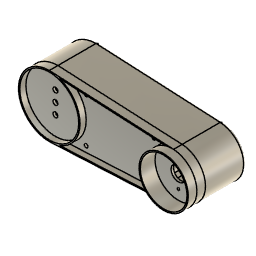
TRARM02_Link3 (Autodesk Fusion 360 design; units mm, degrees)
Autodesk Fusion 360 part; units mm, degrees
sketch "스케치1" plane through (0, 0, 0) normal (0, 0, 1) x (1, 0, 0) in component "TRARM02_Link3A_100x50x7 v1"
  line L0 (19.9753, 100.9938) -> (25, 0)
  line L1 (-19.9753, 100.9938) -> (-25, 0)
  arc A0 (19.9753, 100.9938) -> (-19.9753, 100.9938) centre (0, 100) ccw
  arc A1 (-25, 0) -> (25, 0) centre (0, 0) ccw
  dimension "d1" = 50
  dimension "d222" = 20
  dimension "d223" = 100
  constraint coincident A1.centre origin
  constraint tangent L1 A0
  constraint horizontal A1.centre L1.end
  constraint horizontal A1.centre L0.end
  constraint vertical A1.centre A0.centre
  constraint tangent L0 A0
  measures "d1" diameter of A1
  measures "d222" radius of A0
  measures "d223" distance of A1.centre A0.centre
extrude "돌출1" add sketch "스케치1" along normal blind 2 makes body 1 in component "TRARM02_Link3A_100x50x7 v1"
sketch "스케치2" plane through (0, 0, 2) normal (0, 0, 1) x (-1, 0, 0) in component "TRARM02_Link3A_100x50x7 v1"
  arc A0 (-19.9753, -100.9938) -> (19.9753, -100.9938) centre (0, -100) ccw
  line L0 (19.9753, -100.9938) -> (25, 0)
  line L1 (-25, 0) -> (-19.9753, -100.9938)
  line L2 (19.9753, -100.9938) -> (25, 0)
  arc A1 (-19.9753, -100.9938) -> (19.9753, -100.9938) centre (0, -100) ccw
  line L3 (-25, 0) -> (-19.9753, -100.9938)
  arc A2 (25, 0) -> (-25, 0) centre (0, 0) ccw
  line L4 (-23.5864, -8.2873) -> (-19.2868, -94.7068)
  line L5 (19.2868, -94.7068) -> (23.5864, -8.2873)
  circle A3 centre (0, -100) radius 19
  circle A4 centre (0, 0) radius 23.9691
  arc A5 (-23.5864, -8.2873) -> (23.5864, -8.2873) centre (0, 0) ccw
  arc A6 (25, 0) -> (-25, 0) centre (0, 0) ccw
  arc A7 (-19.9753, -100.9938) -> (19.9753, -100.9938) centre (0, -100) ccw
  arc A8 (19.2868, -94.7068) -> (-19.2868, -94.7068) centre (0, -100) ccw
  constraint concentric A0 A7
  constraint concentric A1 A3
  constraint tangent L4 A3
  constraint concentric A2 A5
  constraint coincident L1.start A5
  constraint concentric A2 A4
  constraint tangent L4 A4
  constraint concentric A5 A6
  constraint coincident L5.start A7
  constraint concentric A7 A8
extrude "돌출25" add sketch "스케치2" along normal blind 5 bodies 1 in component "TRARM02_Link3A_100x50x7 v1"
sketch "스케치22" plane through (0, 0, 2) normal (0, 0, 1) x (-1, 0, 0) in component "TRARM02_Link3A_100x50x7 v1"
  circle A0 centre (0, 0) radius 2
  circle A1 centre (-8.7, 0) radius 2
  circle A2 centre (8.7, 0) radius 2
  circle A3 centre (0, -100) radius 6
  circle A4 centre (-11, -100) radius 1
  circle A5 centre (11, -100) radius 1
  dimension "d208" = 4
  dimension "d209" = 8.7
  dimension "d210" = 8.7
  dimension "d226" = 12
  dimension "d227" = 2
  dimension "d228" = 11
  dimension "d229" = 11
  dimension "d230" = 100
  constraint coincident A0.centre origin
  constraint equal A0 A2
  constraint equal A0 A1
  constraint horizontal A0.centre A1.centre
  constraint horizontal A0.centre A2.centre
  constraint equal A4 A5
  constraint horizontal A3.centre A5.centre
  constraint horizontal A3.centre A4.centre
  constraint vertical A0.centre A3.centre
  measures "d208" diameter of A0
  measures "d209" distance of A0.centre A1.centre
  measures "d210" distance of A0.centre A2.centre
  measures "d226" diameter of A3
  measures "d227" diameter of A4
  measures "d228" distance of A3.centre A4.centre
  measures "d229" distance of A3.centre A5.centre
  measures "d230" distance of A0.centre A3.centre
extrude "돌출26" cut sketch "스케치22" against normal blind 2 bodies 1 in component "TRARM02_Link3A_100x50x7 v1"
sketch "스케치24" plane through (0, 0, 7) normal (0, 0, 1) x (-1, 0, 0) in component "TRARM02_Link3A_100x50x7 v1"
  circle A0 centre (0, -100) radius 20
  circle A1 centre (0, -100) radius 6
  arc A2 (-19.9753, -100.9938) -> (19.9753, -100.9938) centre (0, -100) ccw
  circle A3 centre (0, -100) radius 19
  circle A4 centre (0, -100) radius 19
  constraint concentric A0 A1
  constraint tangent A0 A2
  constraint concentric A1 A3
  constraint tangent A3 A4
extrude "돌출28" add sketch "스케치24" along normal blind 7 contours A0 A2 bodies 1 in component "TRARM02_Link3A_100x50x7 v1"
sketch "스케치23" plane through (0, 0, 2) normal (0, 0, 1) x (-1, 0, 0) in component "TRARM02_Link3A_100x50x7 v1"
  circle A0 centre (-18, -25) radius 1.5
  circle A1 centre (-15, -80) radius 1.5
  circle A2 centre (15, -80) radius 1.5
  circle A3 centre (18, -25) radius 1.5
  circle A4 centre (0, -100) radius 6
  dimension "d214" = 3
  dimension "d215" = 18
  dimension "d216" = 18
  dimension "d217" = 25
  dimension "d225" = 20
  dimension "d233" = 15
  dimension "d234" = 15
  constraint equal A0 A3
  constraint equal A0 A1
  constraint equal A1 A2
  constraint horizontal A1.centre A2.centre
  constraint horizontal A0.centre A3.centre
  measures "d214" diameter of A0
  measures "d215" horizontal distance of origin A0.centre
  measures "d216" horizontal distance of origin A3.centre
  measures "d217" vertical distance of origin A0.centre
  measures "d225" vertical distance of A1.centre A4.centre
  measures "d233" horizontal distance of A1.centre A4.centre
  measures "d234" horizontal distance of A2.centre A4.centre
extrude "돌출27" cut sketch "스케치23" against normal blind 2 contours A0 | A1 | A2 | A3 bodies 1 in component "TRARM02_Link3A_100x50x7 v1"
move_body "이동1" bodies 1 to x (-1, 0, 0) y (0, 1, 0) z (0, 0, -1) at (0, 0, 0) in component "TRARM02_Link3A_100x50x7 v1"
move_body "이동2" bodies 1 to x (1, 0, 0) y (0, 1, 0) z (0, 0, 1) at (0, 0, 7) in component "TRARM02_Link3A_100x50x7 v1"
sketch "스케치1 (2)" plane through (0, 0, 0) normal (0, 0, 1) x (1, 0, 0) in component "TRARM02_Link3B_100x50x33 v1"
  line L0 (19.9753, 100.9938) -> (25, 0)
  line L1 (-19.9753, 100.9938) -> (-25, 0)
  arc A0 (19.9753, 100.9938) -> (-19.9753, 100.9938) centre (0, 100) ccw
  arc A1 (-25, 0) -> (25, 0) centre (0, 0) ccw
  dimension "d1_1" = 50
  dimension "d222_1" = 20
  dimension "d223_1" = 100
  constraint coincident A1.centre origin
  constraint tangent L1 A0
  constraint horizontal A1.centre L1.end
  constraint horizontal A1.centre L0.end
  constraint vertical A1.centre A0.centre
  constraint tangent L0 A0
  measures "d1_1" diameter of A1
  measures "d222_1" radius of A0
  measures "d223_1" distance of A1.centre A0.centre
extrude "돌출1'" add sketch "스케치1 (2)" along normal blind 2 separate body makes body 2 in component "TRARM02_Link3B_100x50x33 v1"
sketch "스케치2 (2)" plane through (0, 0, 2) normal (0, 0, 1) x (-1, 0, 0) in component "TRARM02_Link3B_100x50x33 v1"
  line L0 (19.9753, -100.9938) -> (25, 0)
  arc A0 (-19.9753, -100.9938) -> (19.9753, -100.9938) centre (0, -100) ccw
  line L1 (-25, 0) -> (-19.9753, -100.9938)
  arc A1 (25, 0) -> (-25, 0) centre (0, 0) ccw
  arc A2 (23.9988, 0) -> (-23.9988, 0) centre (0, 0) ccw
  arc A3 (-18.9765, -100.9441) -> (18.9765, -100.9441) centre (0, -100) ccw
  line L2 (-15, -77) -> (-20.1678, -77)
  line L3 (-15, -83) -> (-19.8693, -83)
  line L4 (15, -77) -> (20.1678, -77)
  line L5 (15, -83) -> (19.8693, -83)
  arc A4 (15, -77) -> (15, -83) centre (15, -80) ccw
  line L6 (18.9765, -100.9441) -> (19.8693, -83)
  line L7 (-19.8693, -83) -> (-18.9765, -100.9441)
  arc A5 (-15, -83) -> (-15, -77) centre (-15, -80) ccw
  line L8 (-18, -28) -> (-22.6057, -28)
  line L9 (-18, -22) -> (-22.9042, -22)
  line L10 (18, -28) -> (22.6057, -28)
  line L11 (18, -22) -> (22.9042, -22)
  arc A6 (18, -22) -> (18, -28) centre (18, -25) ccw
  line L12 (20.1678, -77) -> (22.6057, -28)
  line L13 (22.9042, -22) -> (23.9988, 0)
  line L14 (-23.9988, 0) -> (-22.9042, -22)
  line L15 (-22.6057, -28) -> (-20.1678, -77)
  arc A7 (-18, -28) -> (-18, -22) centre (-18, -25) ccw
  dimension "d241" = 6
  dimension "d242" = 15
  dimension "d243" = 15
  dimension "d245" = 25
  dimension "d246" = 18
  dimension "d247" = 18
  dimension "d255" = 20
  constraint equal A6 A7
  constraint equal A5 A7
  constraint equal A4 A5
  constraint horizontal A7.centre A6.centre
  constraint horizontal A5.centre A4.centre
  constraint coincident L2.start A5
  constraint horizontal L2
  constraint coincident L3.end L14
  constraint parallel L2 L3
  constraint coincident L4.start A4
  constraint coincident L4.end L6
  constraint parallel L3 L4
  constraint parallel L4 L5
  constraint coincident L5 A4.end
  constraint coincident L4 A4.start
  constraint concentric A1 A2
  constraint concentric A0 A3
  constraint tangent A3 L14
  constraint tangent A3 L6
  constraint collinear L6 L12
  constraint collinear L7 L14
  constraint coincident L2 A5.end
  constraint vertical A5.centre L2.start
  constraint vertical A5.centre L3.start
  constraint vertical A4.centre L5.start
  constraint vertical A4.centre L4.start
  constraint coincident L5.start A4.end
  constraint coincident L8.end L14
  constraint horizontal L8
  constraint coincident L9.start A7
  constraint parallel L8 L9
  constraint parallel L9 L10
  constraint coincident L11.end L12
  constraint parallel L10 L11
  constraint collinear L12 L13
  constraint collinear L14 L15
  constraint coincident L9 A7.end
  constraint vertical A7.centre L8.start
  constraint vertical A7.centre L9.start
  constraint vertical A6.centre L10.start
  constraint vertical A6.centre L11.start
  constraint horizontal A1.centre A2.end
  measures "d241" diameter of A7
  measures "d242" horizontal distance of A1.centre A5.centre
  measures "d243" horizontal distance of A1.centre A4.centre
  measures "d245" vertical distance of A1.centre A7.centre
  measures "d246" horizontal distance of A1.centre A7.centre
  measures "d247" horizontal distance of A1.centre A6.centre
  measures "d255" vertical distance of A0.centre A5.centre
extrude "돌출29" add sketch "스케치2 (2)" along normal blind 31 bodies 2 in component "TRARM02_Link3B_100x50x33 v1"
sketch "스케치26" plane through (0, 0, 33) normal (0, 0, 1) x (-1, 0, 0) in component "TRARM02_Link3B_100x50x33 v1"
  circle A0 centre (18, -25) radius 1.45
  arc A1 (18, -22) -> (18, -28) centre (18, -25) ccw
  circle A2 centre (-18, -25) radius 1.45
  arc A3 (-18, -28) -> (-18, -22) centre (-18, -25) ccw
  circle A4 centre (15, -80) radius 1.45
  arc A5 (15, -77) -> (15, -83) centre (15, -80) ccw
  circle A6 centre (-15, -80) radius 1.45
  arc A7 (-15, -83) -> (-15, -77) centre (-15, -80) ccw
  dimension "d248" = 2.9
  constraint concentric A0 A1
  constraint concentric A2 A3
  constraint concentric A4 A5
  constraint concentric A6 A7
  constraint equal A4 A6
  constraint equal A0 A6
  constraint equal A0 A2
  measures "d248" diameter of A0
extrude "돌출30" cut sketch "스케치26" against normal blind 5 bodies 2 in component "TRARM02_Link3B_100x50x33 v1"
fillet "필렛6" radius 2 4 edges at (0, -25, 0) (-22.4876, 50.4969, 0) (0, 120, 0) (22.4876, 50.4969, 0) on bodies 2 in component "TRARM02_Link3B_100x50x33 v1"
move_body "이동3" bodies 1 to x (0, -1, 0) y (1, 0, 0) z (0, 0, 1) at (0, 0, 0) in component "TRARM02_Link3A_100x50x7 v1"
move_body "이동1'" bodies 2 to x (0, 1, 0) y (-1, 0, 0) z (0, 0, 1) at (0, 0, 0) in component "TRARM02_Link3B_100x50x33 v1"
move_body "이동2'" bodies 2 to x (1, 0, 0) y (0, 0, 1) z (0, -1, 0) at (0, 40, 40) in component "TRARM02_Link3B_100x50x33 v1"
move_body "이동4" bodies 1 to x (1, 0, 0) y (0, 0, -1) z (0, 1, 0) at (0, 0, 0) in component "TRARM02_Link3A_100x50x7 v1"
component "TRARM02_Link3A_100x50x7 v1" placed x (1, 0, 0) y (0, 1, 0) z (0, 0, 1) at (0, 0, 0)
component "TRARM02_Link3B_100x50x33 v1" placed x (-1, 0, 0) y (0, 1, 0) z (0, 0, -1) at (0, 0, 40)
